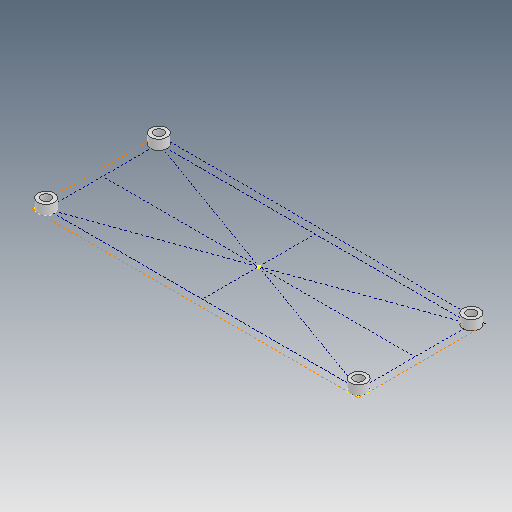
# Autodesk Inventor part: relay_module_standoffs_plate
Saved by Autodesk Inventor 2025.4 (Build 294407020, 407B)
## iProperties
Created: 2026-06-20
Part Number: relay_module_standoffs_plate
Material: Generic
Document SubType Name: Modeling
Designer: Aiden
Density: 1 g/cm^3
Appearance: Default
Author: Aiden
Autodesk Inventor part; units mm, degrees
ref_plane "YZ Plane" through (0, 0, 0) normal (1, 0, 0) x (0, 1, 0)
ref_plane "XZ Plane" through (0, 0, 0) normal (0, 1, 0) x (-1, 0, 0)
ref_plane "XY Plane" through (0, 0, 0) normal (0, 0, 1) x (1, 0, 0)
sketch "Relay Hole Layout" plane through (0, 0, 0) normal (0, 1, 0) x (-1, 0, 0)
  line L0 (64.4668, 23.2607) -> (-64.4668, 23.2607) construction
  line L1 (-64.4668, 23.2607) -> (-64.4668, -23.2607) construction
  line L2 (-64.4668, -23.2607) -> (64.4668, -23.2607) construction
  line L3 (64.4668, -23.2607) -> (64.4668, 23.2607) construction
  line L4 (64.4668, 23.2607) -> (-64.4668, -23.2607) construction
  line L5 (-64.4668, 23.2607) -> (64.4668, -23.2607) construction
  circle A0 centre (64.4668, -23.2607) radius 1.625 construction
  line L6 (0, -23.2607) -> (0, 23.2607) construction
  line L7 (64.4668, 0) -> (-64.4668, 0) construction
  circle A1 centre (-64.4668, -23.2607) radius 1.625 construction
  circle A2 centre (64.4668, 23.2607) radius 1.625 construction
  circle A3 centre (-64.4668, 23.2607) radius 1.625 construction
  line L8 (67.4918, -26.2857) -> (-67.4918, -26.2857) construction
  line L9 (-67.4918, -26.2857) -> (-67.4918, 26.2857) construction
  line L10 (-67.4918, 26.2857) -> (67.4918, 26.2857) construction
  line L11 (67.4918, 26.2857) -> (67.4918, -26.2857) construction
  line L12 (66.0918, -23.2607) -> (67.4918, -23.2607) construction
  line L13 (-64.4668, 24.8857) -> (-64.4668, 26.2857) construction
  line L14 (-66.0918, 23.2607) -> (-67.4918, 23.2607) construction
  point P0 (0, 0)
  dimension "d2" = 3.25
  dimension "d0" = 46.5214
  dimension "d1" = 128.9336
  dimension "d5" = 1.4
  dimension "d6" = 1.4
  dimension "d7" = 1.4
  dimension "d8" = 1.4
  constraints: 30 end point, 6 midpoint, 5 perpendicular, 4 parallel, 3 centre point, 3 point on line, 3 symmetric about line, 2 horizontal, 2 point on circle, 1 coincident, 1 horizontal alignment, 5 other
  measures "d0" distance of L2.end L0.start
  measures "d1" distance of L1.end L2.end
  measures "d6" distance of L12.start L12.end
  measures "d7" distance of L14.start L14.end
  measures "d8" distance of L13.start L13.end
sketch "Sketch2" plane through (0, 0, 0) normal (0, 1, 0) x (-1, 0, 0)
  circle A0 centre (64.4668, -23.2607) radius 1.625 construction
  circle A1 centre (-64.4668, -23.2607) radius 1.625 construction
  circle A2 centre (-64.4668, 23.2607) radius 1.625 construction
  circle A3 centre (64.4668, 23.2607) radius 1.625 construction
  circle A4 centre (64.4668, -23.2607) radius 3.375
  circle A5 centre (-64.4668, -23.2607) radius 3.375
  circle A6 centre (-64.4668, 23.2607) radius 3.375
  circle A7 centre (64.4668, 23.2607) radius 3.375
  point P0 (0, 0)
  dimension "d9" = 1.75
  constraints: 4 centre point, 4 coincident, 3 equal radius
  measures "d9" radial gap between concentric circles of A4 A0
extrude "Extrusion2" add sketch "Sketch2" along normal blind 4
sketch "Sketch3" plane through (-64.4668, 4, -23.2607) normal (0, 1, 0) x (1, 0, 0)
  circle A0 centre (0, 0) radius 3.375 projected
  circle A1 centre (128.9336, 0) radius 3.375 projected
  circle A2 centre (128.9336, -46.5214) radius 3.375 projected
  circle A3 centre (0, -46.5214) radius 3.375 projected
  point P0 (64.4668, -23.2607)
  constraints: 4 coincident
hole "Hole1" at (-64.4668, 4, -23.2607) at (64.4668, 4, -23.2607) at (64.4668, 4, 23.2607) at (-64.4668, 4, 23.2607) direction (0, -1, 0) diameter 4 depth 3
sketch "Sketch4" plane through (-64.4668, 0, -23.2607) normal (0, -1, 0) x (1, 0, 0)
  circle A0 centre (0, 0) radius 2 construction
  circle A1 centre (0, 46.5214) radius 2 construction
  circle A2 centre (128.9336, 46.5214) radius 3.375 construction
  circle A3 centre (128.9336, 0) radius 2 construction
  line L0 (0, 0) -> (128.9336, 0) construction
  circle A4 centre (0, 46.5214) radius 3.375 construction
  line L1 (0, 46.5214) -> (128.9336, 46.5214) construction
  point P0 (64.4668, 23.2607)
  constraints: 4 coincident, 4 end point, 2 horizontal
body "Solid2"
